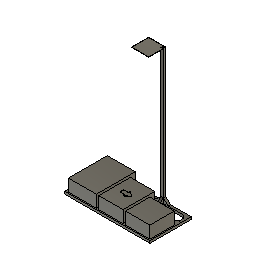
electronics_box (Autodesk Fusion 360 design; units mm, degrees)
Autodesk Fusion 360 part; units mm, degrees
sketch "Sketch1" plane through (0, 0, 0) normal (0, 1, 0) x (1, 0, 0)
  line L0 (350, 170) -> (-350, 170)
  line L1 (-350, 170) -> (-350, -170)
  line L2 (-350, -170) -> (350, -170)
  line L3 (350, -170) -> (350, 170)
  line L4 (350, 170) -> (-350, -170) construction
  line L5 (-350, 170) -> (350, -170) construction
  line L6 (-330, -150) -> (330, -150)
  line L7 (330, -150) -> (330, 150)
  line L8 (330, 150) -> (-330, 150)
  line L9 (-330, 150) -> (-330, -150)
  line L10 (-330, 130) -> (-310, 150)
  line L11 (0, -20) -> (0, -2.5)
  line L12 (330, 130) -> (310, 150)
  line L13 (2.5, 0) -> (20, 0)
  line L14 (-330, -130) -> (-310, -150)
  line L15 (330, -130) -> (310, -150)
  line L16 (-330, 160) -> (-100, 160) construction
  line L17 (-100, 160) -> (-100, -160) construction
  line L18 (-100, -160) -> (-330, -160) construction
  line L19 (-330, -160) -> (-330, 160) construction
  line L20 (-100, 150) -> (-80, 150)
  line L21 (-80, 150) -> (-80, -150)
  line L22 (-80, -150) -> (-100, -150)
  line L23 (-100, -150) -> (-100, 150)
  line L24 (-100, 150) -> (-100, 170) construction
  line L25 (-80, -150) -> (-80, -170) construction
  line L26 (-80, -160) -> (120, -160) construction
  line L27 (120, -160) -> (120, 100) construction
  line L28 (120, 100) -> (-80, 100) construction
  line L29 (-80, 100) -> (-80, -160) construction
  line L30 (120, -150) -> (140, -150)
  line L31 (140, -150) -> (140, 150)
  line L32 (140, 150) -> (120, 150)
  line L33 (120, 150) -> (120, -150)
  line L34 (-80, 100) -> (120, 100)
  line L35 (120, 100) -> (120, 120)
  line L36 (120, 120) -> (-80, 120)
  line L37 (-80, 120) -> (-80, 100)
  line L38 (-60, 100) -> (-80, 80)
  line L39 (100, 120) -> (120, 140)
  line L40 (140, 50) -> (330, 50)
  line L41 (330, 50) -> (330, 70)
  line L42 (330, 70) -> (140, 70)
  line L43 (140, 70) -> (140, 50)
  line L44 (160, 50) -> (140, 30)
  line L45 (310, 70) -> (330, 90)
  line L46 (-120, 150) -> (-100, 130)
  line L47 (-80, -130) -> (-60, -150)
  line L48 (120, -130) -> (100, -150)
  line L49 (140, 130) -> (160, 150)
  dimension "d1" = 700
  dimension "d2" = 340
  dimension "d3" = -20
  dimension "d4" = 20
  dimension "d6" = 20
  dimension "d7" = 230
  dimension "d8" = 320
  dimension "d9" = 20
  dimension "d10" = 230
  dimension "d11" = 200
  dimension "d12" = 260
  dimension "d13" = 20
  dimension "d14" = 300
  dimension "d15" = 200
  dimension "d16" = 20
  dimension "d17" = 20
  dimension "d18" = 20
  dimension "d19" = 20
  dimension "d20" = 20
  dimension "d21" = 20
  dimension "d22" = 200
  dimension "d23" = 20
  dimension "d24" = 20
  dimension "d25" = 20
  dimension "d26" = 20
  dimension "d40" = 20
  dimension "d41" = 20
  dimension "d42" = 20
  dimension "d43" = 20
  dimension "d44" = 20
  dimension "d45" = 20
  dimension "d46" = 20
  dimension "d47" = 20
  constraint horizontal L0
  constraint perpendicular L0 L1
  constraint parallel L0 L2
  constraint parallel L1 L3
  constraint coincident L4 origin
  constraint coincident L5 origin
  constraint coincident L9 L10.start
  constraint coincident L8 L10.end
  constraint symmetric L10.start L11 L12.start
  constraint symmetric L10.end L11 L12.end
  constraint symmetric L10.start L13 L14.start
  constraint symmetric L10.end L13 L14.end
  constraint symmetric L12.start L13 L15.start
  constraint symmetric L12.end L13 L15.end
  constraint horizontal L16
  constraint vertical L17
  constraint horizontal L18
  constraint vertical L19
  constraint horizontal L20
  constraint vertical L21
  constraint horizontal L22
  constraint vertical L23
  constraint coincident L6 L21.end
  constraint coincident L8 L20.start
  constraint coincident L0 L24.end
  constraint perpendicular L0 L24
  constraint midpoint L16.end L24
  constraint coincident L2 L25.end
  constraint perpendicular L2 L25
  constraint horizontal L26
  constraint vertical L27
  constraint horizontal L28
  constraint vertical L29
  constraint midpoint L25 L26.start
  constraint horizontal L30
  constraint vertical L31
  constraint horizontal L32
  constraint vertical L33
  constraint coincident L27 L30.start
  constraint coincident L6 L30.start
  constraint horizontal L34
  constraint vertical L35
  constraint horizontal L36
  constraint vertical L37
  constraint coincident L28 L38.start
  constraint coincident L29 L38.end
  constraint coincident L36 L39.start
  constraint coincident L33 L39.end
  constraint horizontal L40
  constraint vertical L41
  constraint horizontal L42
  constraint vertical L43
  constraint coincident L7 L41.end
  constraint coincident L31 L40.start
  constraint coincident L40 L44.start
  constraint coincident L31 L44.end
  constraint coincident L42 L45.start
  constraint coincident L7 L45.end
  constraint coincident L8 L46.start
  constraint coincident L23 L46.end
  constraint coincident L29 L47.start
  constraint coincident L6 L47.end
  constraint coincident L27 L48.start
  constraint coincident L6 L48.end
  constraint coincident L31 L49.start
  constraint coincident L8 L49.end
  measures "d1" distance of L1.end L2.end
  measures "d2" distance of L0.end L1.end
  measures "d4" distance of L8.end L10.end
  measures "d6" distance of L8.end L10.start
  measures "d7" distance of L16.start L16.end
  measures "d8" distance of L16.start L18.end
  measures "d9" distance of L21 L23
  measures "d10" distance of L9 L23
  measures "d11" distance of L27.end L28.end
  measures "d12" distance of L26.end L27.end
  measures "d13" distance of L30.start L30.end
  measures "d14" distance of L30.start L32.end
  measures "d15" distance of L28.end L27.end
  measures "d16" distance of L28.end L36.end
  measures "d17" distance of L28.end L38.start
  measures "d18" distance of L28.end L38.end
  measures "d19" distance of L35.end L39.start
  measures "d20" distance of L35.end L39.end
  measures "d21" distance of L40 L42
  measures "d22" distance of L6 L40
  measures "d23" distance of L41.end L45.start
  measures "d24" distance of L41.end L45.end
  measures "d25" distance of L40.start L44.start
  measures "d26" distance of L40.start L44.end
  measures "d40" distance of L20.start L46.start
  measures "d41" distance of L20.start L46.end
  measures "d42" distance of L21.end L47.end
  measures "d43" distance of L21.end L47.start
  measures "d44" distance of L30.start L48.end
  measures "d45" distance of L30.start L48.start
  measures "d46" distance of L31.end L49.end
  measures "d47" distance of L31.end L49.start
extrude "Extrude1" add sketch "Sketch1" along normal blind 20 contours L0 L1 L2 L3 | L6 L9 L14 | L6 L8 L20 L21 L22 L23 L37 | L8 L9 L10 | L6 L21 L47 | L8 L23 L46 | L6 L33 L48 | L21 L34 L38 | L6 L8 L30 L31 L32 L33 L35 L43 | L21 L33 L34 L35 L36 L37 | L8 L31 L49 | L33 L36 L39 | L6 L7 L15 | L31 L40 L44 | L7 L31 L40 L41 L42 L43 | L7 L8 L12 | L7 L42 L45
sketch "Sketch2" plane through (0, 20, 0) normal (0, 1, 0) x (-1, 0, 0)
  line L0 (60, -100) -> (-120, -100)
  line L1 (-120, -100) -> (-120, 130)
  line L2 (-100, 150) -> (60, 150)
  line L3 (80, 130) -> (80, -80)
  line L4 (80, -80) -> (60, -100)
  line L5 (80, -150) -> (-120, -150)
  line L6 (-120, -150) -> (-120, -140)
  line L7 (-120, -140) -> (-100, -120)
  line L8 (-100, -120) -> (80, -120)
  line L9 (80, -120) -> (80, -150)
  line L10 (-330, -50) -> (-330, 130)
  line L11 (-330, 130) -> (-310, 150)
  line L12 (-310, 150) -> (-140, 150)
  line L13 (-140, 150) -> (-140, -30)
  line L14 (-140, -30) -> (-160, -50)
  line L15 (-160, -50) -> (-330, -50)
  line L16 (-310, -70) -> (-140, -70)
  line L17 (-140, -70) -> (-140, -130)
  line L18 (-160, -150) -> (-310, -150)
  line L19 (-310, -150) -> (-330, -130)
  line L20 (-330, -130) -> (-330, -90)
  line L21 (-330, -90) -> (-310, -70)
  line L22 (330, 130) -> (330, -130)
  line L23 (330, -130) -> (310, -150)
  line L24 (310, -150) -> (120, -150)
  line L25 (100, -130) -> (100, 150)
  line L26 (100, 150) -> (310, 150)
  line L27 (310, 150) -> (330, 130)
  line L28 (-350, 170) -> (-350, -170)
  line L29 (-350, -170) -> (350, -170)
  line L30 (350, -170) -> (350, 170)
  line L31 (350, 170) -> (-350, 170)
  line L32 (330, 160) -> (100, 160)
  line L33 (100, 160) -> (100, -160)
  line L34 (100, -160) -> (330, -160)
  line L35 (330, -160) -> (330, 160)
  line L36 (80, 160) -> (-120, 160)
  line L37 (-120, 160) -> (-120, -100)
  line L38 (-120, -100) -> (80, -100)
  line L39 (80, -100) -> (80, 160)
  line L40 (-140, 160) -> (-340, 160)
  line L41 (-340, 160) -> (-340, -40)
  line L42 (-340, -40) -> (-140, -40)
  line L43 (-140, -40) -> (-140, 160)
  line L44 (350, 160) -> (-350, 160)
  line L45 (-340, 160) -> (-340, 147.3355)
  line L46 (120, -150) -> (100, -130)
  line L47 (-120, 130) -> (-100, 150)
  line L48 (60, 150) -> (80, 130)
  line L49 (-140, -130) -> (-160, -150)
  dimension "d29" = 200
  dimension "d30" = 200
  dimension "d31" = 200
  dimension "d32" = 260
  dimension "d33" = 230
  dimension "d34" = 320
  dimension "d35" = 10
  dimension "d37" = 10
  constraint horizontal L32
  constraint vertical L33
  constraint horizontal L34
  constraint vertical L35
  constraint horizontal L36
  constraint vertical L37
  constraint horizontal L38
  constraint vertical L39
  constraint horizontal L40
  constraint vertical L41
  constraint horizontal L42
  constraint vertical L43
  constraint coincident L28 L44.end
  constraint perpendicular L28 L44
  constraint coincident L30 L44.start
  constraint coincident L32.start L44
  constraint collinear L22 L35
  constraint collinear L3 L39
  constraint collinear L36 L44
  constraint collinear L40 L44
  constraint coincident L44 L40.end
  constraint perpendicular L44 L45
  constraint collinear L41 L45
  measures "d29" distance of L40.end L41.end
  measures "d30" distance of L40.start L40.end
  measures "d31" distance of L36.start L36.end
  measures "d32" distance of L36.start L38.end
  measures "d33" distance of L32.start L32.end
  measures "d34" distance of L32.start L34.end
  measures "d35" distance of L31 L44.end
  measures "d37" distance of L28 L45
extrude "Extrude2" add sketch "Sketch2" along normal blind 100 contours L0 L1 L2 L3 L4 L37 L38 L39 L47 L48 | L4 L38 L39 | L2 L36 L37 L39 L44 L47 L48 | L10 L11 L12 L40 L41 L42 L43 L44 L45 | L26 L27 L32 L33 L35 L44 | L10 L11 L12 L13 L14 L42 L43 | L22 L23 L24 L25 L26 L27 L33 L35 L46 | L14 L42 L43 | L23 L24 L33 L34 L35 L46
sketch "Sketch5" plane through (0, 120, 0) normal (0, 1, 0) x (-1, 0, 0)
  line L0 (80, -100) -> (80, 160)
  line L1 (80, 160) -> (-120, 160)
  line L2 (-120, 160) -> (-120, -100)
  line L3 (-120, -100) -> (80, -100)
  line L4 (-120, -100) -> (80, 160) construction
  line L5 (-120, 160) -> (80, -100) construction
  line L6 (20, 45) -> (-60, 45)
  line L7 (-60, 45) -> (-60, 15)
  line L8 (-60, 15) -> (20, 15)
  line L9 (20, 15) -> (20, 45)
  line L10 (20, 45) -> (-60, 15) construction
  line L11 (-60, 45) -> (20, 15) construction
  line L12 (-60, 30) -> (-20, 0)
  line L13 (-20, 0) -> (-20, 60)
  line L14 (-20, 60) -> (-60, 30)
  point P0 (-20, 30)
  dimension "d57" = 80
  dimension "d58" = 30
  dimension "d59" = 60
  constraint coincident L2.end L3.start
  constraint coincident L0.end L1.start
  constraint coincident L1.end L2.start
  constraint coincident L0.start L3.end
  constraint horizontal L6
  constraint perpendicular L6 L7
  constraint parallel L6 L8
  constraint parallel L7 L9
  constraint coincident L10 P0
  constraint coincident L11 P0
  constraint midpoint L4 P0
  constraint midpoint L7 L12.start
  constraint perpendicular L6 L13
  constraint coincident P0 L13
  measures "d57" distance of L7.end L8.end
  measures "d58" distance of L6.end L7.end
  measures "d59" distance of L12.end L13.end
extrude "Extrude5" cut sketch "Sketch5" against normal blind 2 contours L6 L8 L9 L13 | L6 L8 L12 L13 L14 | L6 L13 L14 | L8 L12 L13
sketch "Sketch3" plane through (0, 20, 0) normal (0, 1, 0) x (-1, 0, 0)
  line L0 (-330, -50) -> (-330, -40)
  line L1 (-150, -40) -> (-160, -50)
  line L2 (-160, -50) -> (-330, -50)
  line L3 (80, -150) -> (-120, -150)
  line L4 (-120, -150) -> (-120, -140)
  line L5 (-120, -140) -> (-100, -120)
  line L6 (-100, -120) -> (80, -120)
  line L7 (80, -120) -> (80, -150)
  line L8 (-330, -90) -> (-310, -70)
  line L9 (-310, -70) -> (-140, -70)
  line L10 (-140, -70) -> (-140, -130)
  line L11 (-140, -130) -> (-160, -150)
  line L12 (-160, -150) -> (-310, -150)
  line L13 (-310, -150) -> (-330, -130)
  line L14 (-330, -130) -> (-330, -90)
  line L15 (-350, 170) -> (-350, -170)
  line L16 (-350, -170) -> (350, -170)
  line L17 (350, -170) -> (350, 170)
  line L18 (350, 170) -> (-350, 170)
  line L19 (-120, -150) -> (-140, -150)
  line L20 (-140, -150) -> (-140, -170)
  line L21 (-140, -170) -> (-120, -170)
  line L22 (-120, -170) -> (-120, -150)
  line L23 (-140, -40) -> (-150, -40)
  line L24 (-330, -40) -> (-340, -40)
  line L25 (-340, -40) -> (-340, 160)
  line L26 (-340, 160) -> (-140, 160)
  line L27 (-140, 160) -> (-140, 150)
  line L28 (-140, 150) -> (-140, -30)
  line L29 (-140, -30) -> (-140, -40)
  line L30 (-120, 130) -> (-120, 160)
  line L31 (-120, 160) -> (80, 160)
  line L32 (80, 160) -> (80, 130)
  line L33 (80, 130) -> (80, -80)
  line L34 (80, -80) -> (80, -100)
  line L35 (80, -100) -> (60, -100)
  line L36 (60, -100) -> (-120, -100)
  line L37 (-120, -100) -> (-120, 130)
  line L38 (100, 150) -> (100, 160)
  line L39 (100, 160) -> (330, 160)
  line L40 (330, 160) -> (330, 130)
  line L41 (330, 130) -> (330, -130)
  line L42 (330, -130) -> (330, -160)
  line L43 (330, -160) -> (100, -160)
  line L44 (100, -160) -> (100, -130)
  line L45 (100, -130) -> (100, 150)
  dimension "d48" = 20
  dimension "d49" = 20
  constraint horizontal L19
  constraint vertical L20
  constraint horizontal L21
  constraint vertical L22
  constraint coincident L3.end L4.start
  measures "d48" distance of L3.end L19.end
  measures "d49" distance of L3.end L21.end
extrude "Extrude3" add sketch "Sketch3" along normal blind 1100 contours L16 L19 L20 L21 L22
sketch "Sketch4" plane through (0, 1120, 0) normal (0, 1, 0) x (-1, 0, 0)
  line L0 (-120, -170) -> (-120, -150)
  line L1 (-120, -150) -> (-140, -150)
  line L2 (-140, -150) -> (-140, -170)
  line L3 (-140, -170) -> (-120, -170)
  line L4 (-140, -170) -> (0, -170)
  line L5 (0, -170) -> (0, -30)
  line L6 (0, -30) -> (-140, -30)
  line L7 (-140, -30) -> (-140, -170)
  line L8 (-120, -150) -> (-140, -170)
  circle A0 centre (-130, -160) radius 2.5
  dimension "d52" = 140
  dimension "d53" = 140
  dimension "d54" = 5
  constraint horizontal L4
  constraint vertical L5
  constraint horizontal L6
  constraint vertical L7
  constraint coincident L2.end L3.start
  constraint coincident L0.end L1.start
  constraint midpoint L8 A0.centre
  measures "d52" distance of L2.end L4.end
  measures "d53" distance of L2.end L6.end
  measures "d54" diameter of A0
extrude "Extrude4" add sketch "Sketch4" along normal blind 3 contours L0 L3 L4 L8 A0 | L0 L1 L4 L5 L6 L7 | L1 L2 L7 L8 A0
move_body "Move1" bodies 1 to x (1, 0, 0) y (0, 0, 1) z (0, -1, 0) at (0, 0, 0)
sketch "Sketch6" plane through (0, 170, 0) normal (0, 1, 0) x (-1, 0, 0)
  line L0 (-350, 0) -> (350, 0)
  line L1 (350, 0) -> (350, 20)
  line L2 (350, 20) -> (-120, 20)
  line L3 (-120, 20) -> (-120, 1120)
  line L4 (-120, 1120) -> (0, 1120)
  line L5 (0, 1120) -> (0, 1123)
  line L6 (0, 1123) -> (-140, 1123)
  line L7 (-140, 1123) -> (-140, 20)
  line L8 (-140, 20) -> (-350, 20)
  line L9 (-350, 20) -> (-350, 0)
  line L10 (-80, 20) -> (-120, 60)
  line L11 (-140, 60) -> (-180, 20)
  dimension "d63" = 40
  dimension "d64" = 40
  dimension "d65" = 40
  dimension "d66" = 40
  constraint coincident L2 L10.start
  constraint coincident L3 L10.end
  constraint coincident L7 L11.start
  constraint coincident L8 L11.end
  measures "d63" distance of L2.end L10.start
  measures "d64" distance of L7.end L11.end
  measures "d65" distance of L7.end L11.start
  measures "d66" distance of L2.end L10.end
extrude "Extrude6" add sketch "Sketch6" against normal blind 20 contours L7 L8 L11 | L2 L3 L10
sketch "Sketch7" plane through (140, 0, 0) normal (1, 0, 0) x (0, 0, -1)
  line L0 (-60, 150) -> (-60, 170)
  line L1 (-60, 170) -> (-1123, 170)
  line L2 (-1123, 170) -> (-1123, 30)
  line L3 (-1123, 30) -> (-1120, 30)
  line L4 (-1120, 30) -> (-1120, 150)
  line L5 (-1120, 150) -> (-60, 150)
  line L6 (-60, 150) -> (-20, 110)
  line L7 (-20, -170) -> (-20, 170)
  line L8 (-20, 150) -> (-60, 150)
  point P0 (-20, 150)
  dimension "d69" = 40
  constraint coincident L0.start L5.end
  constraint coincident L6.end L7
  measures "d69" distance of L6.end P0
extrude "Extrude7" add sketch "Sketch7" against normal blind 20 contours L6 L7 L8
scale "Scale1" factor 0.1 about (0, 0, 0) bodies 1
scale "Scale2" factor 0.01 about (0, 0, 0) bodies 1
